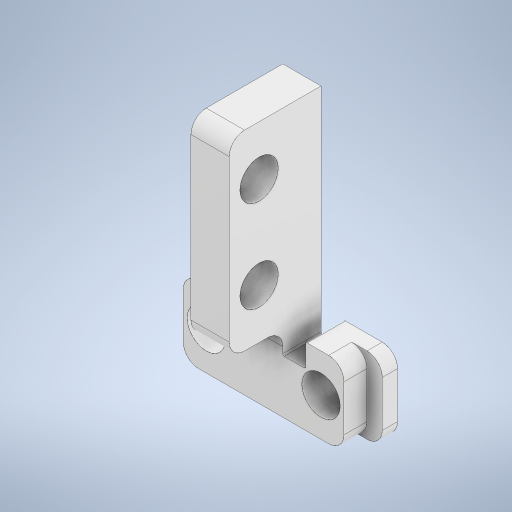
# Autodesk Inventor part: BP_BOX-Support-Bar-Connect1-20
Saved by Autodesk Inventor 2024.3 (Build 283343000, 343)
## iProperties
Created: 2025-11-18
Part Number: BP_BOX-Support-Bar-Connect1-20
Material: ABS プラスチック
Document SubType Name: Modeling
Designer: 佐藤智貴
Density: 1.06 g/cm^3
Appearance: 滑らか - 白
Author: 佐藤智貴
Autodesk Inventor part; units mm, degrees
ref_plane "YZ Plane" through (0, 0, 0) normal (1, 0, 0) x (0, 1, 0)
ref_plane "XZ Plane" through (0, 0, 0) normal (0, 1, 0) x (-1, 0, 0)
ref_plane "XY Plane" through (0, 0, 0) normal (0, 0, 1) x (1, 0, 0)
sketch "スケッチ6" plane through (0, 0, 0) normal (0, 0, 1) x (1, 0, 0)
  line L0 (0, 0) -> (25, 0)
  line L1 (25, 0) -> (25, 30)
  line L2 (25, 30) -> (0, 30)
  line L3 (0, 30) -> (0, 0)
  circle A0 centre (5, 5) radius 2.5
  circle A1 centre (20, 5) radius 2.5
  dimension "d39" = 5
  dimension "d40" = 5
  dimension "d41" = 5
  dimension "d42" = 5
  dimension "d43" = 15
  dimension "d44" = 5
  dimension "d45" = 5
  dimension "d46" = 30
  constraints: 8 end point, 2 centre point, 2 parallel, 1 horizontal, 1 perpendicular
  measures "d39" diameter of A0
  measures "d40" diameter of A1
  measures "d41" distance from line of L0 A0.centre
  measures "d42" distance from line of L0 A1.centre
  measures "d43" distance of A1.centre A0.centre
  measures "d44" distance from line of L3 A0.centre
  measures "d45" distance from line of L1 A1.centre
  measures "d46" distance of L0.end L1.end
extrude "押し出し4" add sketch "スケッチ6" along normal blind 5
sketch "スケッチ7" plane through (0, 0, 5) normal (0, 0, 1) x (1, 0, 0)
  line L0 (25, 30) -> (0, 30) projected
  line L1 (10, 30) -> (15, 30)
  line L2 (15, 30) -> (15, 10)
  line L3 (15, 10) -> (10, 10)
  line L4 (10, 10) -> (10, 30)
  line L5 (25, 0) -> (25, 30) projected
  line L6 (0, 30) -> (0, 0) projected
  line L7 (0, 0) -> (25, 0) projected
  line L8 (10, 30) -> (15, 30)
  line L9 (15, 30) -> (15, 35)
  line L10 (15, 35) -> (10, 35)
  line L11 (10, 35) -> (10, 30)
  dimension "d49" = 5
  dimension "d50" = 10
  dimension "d51" = 10
  dimension "d52" = 10
  dimension "d55" = 5
  dimension "d56" = 5
  constraints: 16 end point, 4 parallel, 2 horizontal, 2 perpendicular, 1 point on line
  measures "d49" distance between parallel lines of L4 L2
  measures "d50" distance between parallel lines of L5 L2
  measures "d51" distance between parallel lines of L6 L4
  measures "d52" distance between parallel lines of L7 L3
  measures "d55" distance between parallel lines of L0 L10
  measures "d56" distance of L9.end L10.end
extrude "押し出し5" add sketch "スケッチ7" along normal blind 10 contours L2 L3 L4 L0 | L0 L11 L10 L9
sketch "スケッチ8" plane through (10, 30, 5) normal (-1, 0, 0) x (0, 0, 1)
  line L0 (10, 5) -> (10, -20) projected
  line L1 (0, 5) -> (10, 5) projected
  line L2 (0, -20) -> (10, -20) projected
  point P0 (-5, -30)
  point P1 (3.1, -13.5)
  point P2 (3.1, -1.5)
  dimension "d57" = 6.9
  dimension "d58" = 6.9
  dimension "d59" = 12
  dimension "d60" = 6.5
  dimension "d61" = 6.5
  measures "d57" distance from line of L0 point (3.1, -13.5)
  measures "d58" distance from line of L0 point (3.1, -1.5)
  measures "d59" distance of point (3.1, -13.5) point (3.1, -1.5)
  measures "d60" distance from line of L1 point (3.1, -1.5)
  measures "d61" distance from line of L2 point (3.1, -13.5)
hole "穴3" at (10, 16.5, 8.1) at (10, 28.5, 8.1) direction (1, 0, 0) diameter 5 depth 8
sketch "スケッチ9" plane through (0, 0, 5) normal (0, 0, 1) x (1, 0, 0)
  line L0 (10, 30) -> (0, 30) projected
  line L1 (0, 30) -> (7, 30)
  line L2 (7, 30) -> (7, 10)
  line L3 (7, 10) -> (0, 10)
  line L4 (0, 10) -> (0, 30)
  line L5 (25, 0) -> (25, 30) projected
  line L6 (25, 30) -> (18, 30)
  line L7 (18, 30) -> (18, 10)
  line L8 (18, 10) -> (25, 10)
  line L9 (25, 10) -> (25, 30)
  point P0 (0, 0)
  point P1 (5, 30)
  point P2 (18, 20)
  point P3 (7, 20)
  dimension "d70" = 20
  dimension "d72" = 7
  dimension "d73" = 7
  constraints: 16 end point, 4 parallel, 3 midpoint, 2 horizontal, 2 perpendicular, 1 point on line
  measures "d70" distance from line of point (5, 30) L3
  measures "d72" distance between parallel lines of L4 L2
  measures "d73" distance between parallel lines of L5 L7
extrude "押し出し6" cut sketch "スケッチ9" against normal blind 10
sketch "スケッチ10" plane through (0, 0, 5) normal (0, 0, 1) x (1, 0, 0)
  line L0 (10, 30) -> (7, 30) projected
  line L1 (7, 30) -> (7, 10) projected
  line L2 (7, 10) -> (0, 10) projected
  line L3 (0, 10) -> (0, 0) projected
  line L4 (0, 0) -> (25, 0) projected
  line L5 (25, 0) -> (25, 10) projected
  line L6 (25, 10) -> (18, 10) projected
  line L7 (18, 10) -> (18, 30) projected
  line L8 (18, 30) -> (15, 30) projected
  circle A0 centre (5, 5) radius 2.5 projected
  circle A1 centre (20, 5) radius 2.5 projected
  line L9 (2, 8) -> (23, 8)
  line L10 (23, 8) -> (23, 2)
  line L11 (23, 2) -> (2, 2)
  line L12 (2, 2) -> (2, 8)
  line L13 (2, 10) -> (2, 0)
  line L14 (24, 10) -> (19, 10) projected
  line L15 (23, 10) -> (23, 0)
  line L16 (15, 30) -> (15, 10) projected
  line L17 (15, 10) -> (10, 10) projected
  line L18 (10, 10) -> (10, 30) projected
  point P0 (2, 2)
  point P1 (23, 2)
  dimension "d77" = 2
  dimension "d78" = 2
  dimension "d79" = 2
  dimension "d80" = 2
  constraints: 12 end point, 4 point on line, 2 parallel, 2 perpendicular, 1 horizontal, 1 vertical
  measures "d77" distance between parallel lines of L4 L11
  measures "d78" distance between parallel lines of L2 L9
  measures "d79" distance between parallel lines of L3 L12
  measures "d80" distance between parallel lines of L5 L10
extrude "押し出し7" cut sketch "スケッチ10" against normal blind 4 contours L18 L17 L16 L8 L7 L6 L15 L9 L13 L2 L1 L0 | L13 L12 L4 L3 L2 | L9 L10 L11 L12 | L15 L6 L5 L4 L10 | L11 L15 L4 L13 | A0 | A1
sketch "スケッチ11" plane through (0, 0, 1) normal (0, 0, 1) x (1, 0, 0)
  line L0 (0, 10) -> (0, 0) projected
  line L1 (25, 0) -> (25, 10) projected
  line L2 (0, 10) -> (25, 10)
  line L3 (25, 10) -> (25, 0)
  line L4 (25, 0) -> (0, 0)
  line L5 (0, 0) -> (0, 10)
  constraints: 8 end point, 2 parallel, 1 horizontal, 1 perpendicular
extrude "押し出し8" add sketch "スケッチ11" along normal blind 4
sketch "スケッチ12" plane through (0, 0, 5) normal (0, 0, 1) x (1, 0, 0)
  circle A0 centre (5, 5) radius 2.5 projected
  circle A1 centre (20, 5) radius 2.5 projected
  point P0 (0, 0)
  constraints: 2 coincident
hole "穴4" at (5, 5, 5) at (20, 5, 5) direction (0, 0, -1) diameter 5 depth 8
sketch "スケッチ13" plane through (10, 30, 5) normal (-1, 0, 0) x (0, 0, 1)
  line L0 (10, -20) -> (10, 5) projected
  line L1 (0, -20) -> (10, -20) projected
  line L2 (10, 5) -> (7, 5)
  line L3 (7, 5) -> (7, -20)
  line L4 (7, -20) -> (10, -20)
  line L5 (10, -20) -> (10, 5)
  line L6 (-4, 0) -> (-4, -20) projected
  line L7 (-4, -20) -> (-1, -20)
  line L8 (-1, -20) -> (-1, 5)
  line L9 (-1, 5) -> (-4, 5)
  line L10 (-4, 5) -> (-4, -20)
  point P0 (-5, -30)
  dimension "d93" = 3
  dimension "d94" = 3
  constraints: 16 end point, 4 parallel, 2 horizontal, 2 perpendicular, 2 point on line
  measures "d93" distance between parallel lines of L0 L3
  measures "d94" distance between parallel lines of L6 L8
extrude "押し出し9" cut sketch "スケッチ13" against normal through all contours L1 L3 L2 L0
sketch "スケッチ14" plane through (10, 30, 5) normal (0, 1, 0) x (1, 0, 0)
  line L0 (5, 4) -> (8, 4) projected
  line L1 (8, 4) -> (8, 5) projected
  line L2 (8, 5) -> (-3, 5) projected
  line L3 (-3, 5) -> (-3, 4) projected
  line L4 (-3, 4) -> (0, 4) projected
  line L5 (0, 4) -> (0, 0) projected
  line L6 (5, 0) -> (0, 0) projected
  line L7 (5, 0) -> (5, 4) projected
  point P0 (-10, 5)
extrude "押し出し10" add sketch "スケッチ14" along normal blind 5
sketch "スケッチ15" plane through (0, 0, 1) normal (0, 0, 1) x (1, 0, 0)
  line L0 (7, 10) -> (10, 10) projected
  line L1 (10, 35) -> (10, 10) projected
  line L2 (7, 35) -> (10, 35) projected
  line L3 (7, 10) -> (7, 35) projected
  line L4 (15, 10) -> (18, 10) projected
  line L5 (18, 35) -> (18, 10) projected
  line L6 (15, 35) -> (18, 35) projected
  line L7 (15, 10) -> (15, 35) projected
  point P0 (0, 0)
extrude "押し出し11" add sketch "スケッチ15" along normal blind 3
sketch "スケッチ16" plane through (0, 0, 5) normal (0, 0, 1) x (1, 0, 0)
  line L0 (25, 0) -> (25, 10) projected
  line L1 (10, 10) -> (0, 10) projected
  line L2 (25, 10) -> (15, 10) projected
  line L3 (10, 10) -> (15, 10) projected
  line L4 (0, 10) -> (0, 0) projected
  line L5 (0, 0) -> (25, 0) projected
  circle A0 centre (20, 5) radius 2.5 projected
  circle A1 centre (5, 5) radius 2.5 projected
  line L6 (2, 10) -> (2, 0)
  line L7 (23, 10) -> (23, 0)
  point P0 (23, 0)
  point P1 (2, 0)
  constraints: 4 end point, 1 parallel
extrude "押し出し12" cut sketch "スケッチ16" against normal blind 3 contours L5 L7 L2 L0 | L5 L4 L1 L6
fillet "フィレット7" radius 2 4 edges at (2, 10, 3.5) (2, 0, 3.5) (23, 10, 3.5) (23, 0, 3.5)
sketch "スケッチ17" plane through (0, 0, 4) normal (0, 0, 1) x (1, 0, 0)
  line L0 (10, 35) -> (10, 10) projected
  line L1 (10, 35) -> (7, 35) projected
  line L2 (7, 35) -> (7, 10) projected
  line L3 (18, 10) -> (18, 35) projected
  line L4 (18, 35) -> (15, 35) projected
  line L5 (15, 10) -> (15, 35) projected
  line L6 (18, 10) -> (15, 10) projected
  line L7 (10, 10) -> (7, 10) projected
  point P0 (0, 0)
extrude "押し出し13" cut sketch "スケッチ17" against normal through all
sketch "スケッチ18" plane through (0, 0, 5) normal (0, 0, 1) x (1, 0, 0)
  line L0 (10, 10) -> (4, 10) projected
  line L1 (10, 10) -> (7, 10)
  line L2 (7, 10) -> (7, 7)
  line L3 (7, 7) -> (10, 7)
  line L4 (10, 7) -> (10, 10)
  line L5 (21, 10) -> (15, 10) projected
  line L6 (15, 10) -> (18, 10)
  line L7 (18, 10) -> (18, 7)
  line L8 (18, 7) -> (15, 7)
  line L9 (15, 7) -> (15, 10)
  point P0 (0, 0)
  dimension "d107" = 3
  dimension "d108" = 3
  dimension "d109" = 3
  constraints: 16 end point, 4 parallel, 2 horizontal, 2 perpendicular, 1 point on line
  measures "d107" distance of L2.end L3.end
  measures "d108" distance of L7.end L8.end
  measures "d109" distance of L6.end L7.end
extrude "押し出し14" cut sketch "スケッチ18" against normal blind 10
fillet "フィレット8" radius 0.2 6 edges at (7, 10, 2.5) (7, 7, 2.5) (18, 10, 2.5) (15, 7, 2.5) (10, 7, 2.5) (18, 7, 2.5)
fillet "フィレット9" radius 2 7 edges at (0, 10, 1) (0, 0, 1) (12.5, 35, 12) (12.5, 10, 12) (12.5, 10, 5) (25, 10, 1) (25, 0, 1)
equation "\"d42\" = d41"
equation "\"d45\" = d44"
equation "\"d58\" = d57"
equation "\"d73\" = d72"
equation "\"d94\" = d93"
equation "\"d108\" = d107"
